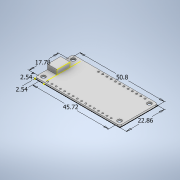
# Autodesk Inventor part: Adafruit Feather 32u4
Saved by Autodesk Inventor 2020.2 (Build 242310000, 310)
## iProperties
Created: 2019-11-22
Part Number: Adafruit Feather 32u4
Material: Generic
Document SubType Name: Sheet Metal
Designer: athiy
Density: 1 g/cm^3
Sheet Metal Rule: Default
Appearance: Default
Author: athiy
Autodesk Inventor part; units mm, degrees
ref_plane "YZ Plane" through (0, 0, 0) normal (1, 0, 0) x (0, 1, 0)
ref_plane "XZ Plane" through (0, 0, 0) normal (0, 1, 0) x (-1, 0, 0)
ref_plane "XY Plane" through (0, 0, 0) normal (0, 0, 1) x (1, 0, 0)
sketch "Sketch1" plane through (0, 0, 0) normal (0, 1, 0) x (-1, 0, 0)
  line L0 (0, 0) -> (-50.8, 0)
  line L1 (-50.8, 0) -> (-50.8, -22.86)
  line L2 (-50.8, -22.86) -> (0, -22.86)
  line L3 (0, -22.86) -> (0, 0)
  line L4 (0, 0) -> (-2.54, 0)
  line L5 (-2.54, 0) -> (-48.26, 0)
  line L6 (0, 0) -> (0, -2.54)
  line L7 (0, -2.54) -> (0, -20.32)
  dimension "d0" = 50.8
  dimension "d1" = 22.86
  dimension "d2" = 2.54
  dimension "d3" = 45.72
  dimension "d4" = 2.54
  dimension "d5" = 17.78
  constraints: 16 end point, 4 point on line, 2 parallel, 1 horizontal, 1 perpendicular
  measures "d0" distance of L2.end L1.end
  measures "d1" distance of L1.end L0.end
  measures "d2" distance of L0.start L4.end
  measures "d3" distance of L4.end L5.end
  measures "d4" distance of L0.start L6.end
  measures "d5" distance of L6.end L7.end
sketch "Sketch2" plane through (0, 0, 0) normal (0, 1, 0) x (-1, 0, 0)
  point P0 (0, 0)
sketch "Sketch3" plane through (0, 0, 0) normal (0, 1, 0) x (-1, 0, 0)
  line L0 (0, -1.27) -> (0, -1.27)
  line L1 (0, -2.504) -> (-2.54, -2.504)
  line L2 (-2.54, -2.504) -> (-2.54, 0)
  line L3 (0, -11.43) -> (-50.8, -11.43)
  circle A0 centre (-2.54, -2.504) radius 1.27
  circle A1 centre (-2.54, -20.356) radius 1.27
  line L4 (-25.4, 0) -> (-25.4, -22.86)
  circle A2 centre (-48.26, -2.504) radius 1.27
  circle A3 centre (-48.26, -20.356) radius 1.27
  line L5 (-1.27, 0) -> (-1.27, 0)
  arc A4 (0, -1.27) -> (-1.27, 0) centre (-1.27, -1.27) ccw
  arc A5 (-1.27, -22.86) -> (0, -21.59) centre (-1.27, -21.59) ccw
  arc A6 (-49.53, 0) -> (-50.8, -1.27) centre (-49.53, -1.27) ccw
  arc A7 (-50.8, -21.59) -> (-49.53, -22.86) centre (-49.53, -21.59) ccw
  line L6 (-25.4, -1.27) -> (-6.35, -1.27)
  line L7 (-25.4, -1.27) -> (-44.45, -1.27)
  circle A8 centre (-6.35, -1.27) radius 0.51
  line L8 (-6.35, -1.27) -> (-8.89, -1.27)
  line L9 (-6.35, -1.27) -> (-3.81, -1.27) construction
  circle A9 centre (-8.89, -1.27) radius 0.51
  circle A10 centre (-8.89, -1.27) radius 0.51
  circle A11 centre (-11.43, -1.27) radius 0.51
  circle A12 centre (-13.97, -1.27) radius 0.51
  circle A13 centre (-16.51, -1.27) radius 0.51
  circle A14 centre (-19.05, -1.27) radius 0.51
  circle A15 centre (-21.59, -1.27) radius 0.51
  circle A16 centre (-24.13, -1.27) radius 0.51
  circle A17 centre (-44.45, -1.27) radius 0.51
  circle A18 centre (-41.91, -1.27) radius 0.51
  circle A19 centre (-39.37, -1.27) radius 0.51
  circle A20 centre (-36.83, -1.27) radius 0.51
  circle A21 centre (-34.29, -1.27) radius 0.51
  circle A22 centre (-31.75, -1.27) radius 0.51
  circle A23 centre (-29.21, -1.27) radius 0.51
  circle A24 centre (-26.67, -1.27) radius 0.51
  circle A25 centre (-16.51, -21.59) radius 0.51
  circle A26 centre (-19.05, -21.59) radius 0.51
  circle A27 centre (-21.59, -21.59) radius 0.51
  circle A28 centre (-24.13, -21.59) radius 0.51
  circle A29 centre (-29.21, -21.59) radius 0.51
  circle A30 centre (-26.67, -21.59) radius 0.51
  circle A31 centre (-31.75, -21.59) radius 0.51
  circle A32 centre (-34.29, -21.59) radius 0.51
  circle A33 centre (-36.83, -21.59) radius 0.51
  circle A34 centre (-39.37, -21.59) radius 0.51
  circle A35 centre (-41.91, -21.59) radius 0.51
  circle A36 centre (-44.45, -21.59) radius 0.51
  line L10 (-1.27, -22.86) -> (-49.53, -22.86)
  line L11 (-50.8, -21.59) -> (-50.8, -1.27)
  line L12 (-49.53, 0) -> (-1.27, 0)
  line L13 (0, -1.27) -> (0, -21.59)
  point P0 (0, 0)
  dimension "d11" = 22.86
  dimension "d12" = 1.27
  dimension "d13" = 19.05
  dimension "d18" = 1.02
  dimension "d19" = 2.54
  dimension "d20" = 180
  dimension "d21" = 1.02
  dimension "d24" = 2.54
  dimension "d31" = 2.54
  dimension "d38" = 2.54
  constraints: 37 centre point, 33 symmetric about line, 28 end point, 8 horizontal, 8 point on circle, 4 perpendicular, 3 point on line, 3 tangent, 2 coincident, 2 collinear, 2 vertical, 40 other
  measures "d11" distance of L4.start L4.end
  measures "d12" radius of A4
  measures "d13" distance of L6.start L6.end
  measures "d18" diameter of A8
  measures "d19" distance of L8.start L8.end
  measures "d20" angle of L8 L9
  measures "d21" diameter of A9
  measures "d24" distance of L8.start A10.centre
  measures "d31" distance of A11.centre A12.centre
  measures "d38" distance of A15.centre A16.centre
sketch "Sketch4" plane through (0, 0, 0) normal (0, 1, 0) x (-1, 0, 0)
  point P0 (0, 0)
extrude "Extrusion1" add sketch "Sketch3" along normal blind 1.016 contours L13 L3 L4 L12 L2 A0 L1 | L1 A0 L2 L12 A4 L13 | L13 A5 L10 L4 L3 | L4 L10 A7 L11 L3 | L3 L11 A6 L12 L4
sketch "Sketch5" plane through (0, 1.016, 0) normal (0, 1, 0) x (1, 0, 0)
  line L0 (0, 21.59) -> (0, 1.27) projected
  line L1 (0, 11.43) -> (0, 15.38)
  line L2 (0, 15.38) -> (5.6, 15.38)
  line L3 (5.6, 15.38) -> (5.6, 7.48)
  line L4 (5.6, 7.48) -> (0, 7.48)
  point P0 (0, 0)
  dimension "d46" = 3.95
  dimension "d49" = 5.6
  dimension "d50" = 7.9
  constraints: 8 end point, 2 perpendicular, 2 point on line, 1 horizontal, 1 midpoint
  measures "d46" distance of L1.start L1.end
  measures "d49" distance of L1.end L2.end
  measures "d50" distance of L2.end L3.end
extrude "Extrusion2" add sketch "Sketch5" along normal blind 2.8
sketch "Sketch6" plane through (5.6, 1.016, -7.48) normal (1, 0, 0) x (0, 0, -1)
  line L0 (0, 0) -> (0, 2.8) projected
  line L1 (7.9, 2.8) -> (0, 2.8) projected
  line L2 (7.9, 0) -> (7.9, 2.8) projected
  line L3 (-6.21, 0) -> (14.11, 0) projected
  point P0 (-7.48, -1.016)
sketch "Sketch7" plane through (0, 0, -21.59) normal (-1, 0, 0) x (0, 0, 1)
  line L0 (6.21, 3.816) -> (6.51, 3.816)
  line L1 (6.51, 3.216) -> (13.81, 3.216)
  line L2 (13.81, 3.216) -> (13.81, 1.316)
  line L3 (13.81, 1.316) -> (6.51, 1.316)
  line L4 (6.51, 1.316) -> (6.51, 3.216)
  point P0 (21.59, 0)
  dimension "d61" = 0.3
  dimension "d62" = 0.6
  dimension "d63" = 7.3
  dimension "d64" = 1.9
  constraints: 10 end point, 3 perpendicular
  measures "d61" distance of L0.start L0.end
  measures "d62" distance of L0.end L1.start
  measures "d63" distance of L1.start L1.end
  measures "d64" distance of L1.end L2.end
sketch "Sketch8" plane through (5.6, 1.016, -7.48) normal (1, 0, 0) x (0, 0, -1)
  point P0 (-7.48, -1.016)
extrude "Extrusion3" cut sketch "Sketch7" against normal blind 2.15
equation "\"BendRadius\" = Thickness"
equation "\"BendReliefWidth\" = Thickness"
equation "\"BendReliefDepth\" = 0.5 * Thickness"
equation "\"CornerReliefSize\" = 4 * Thickness"
equation "\"MinimumRemnant\" = 2 * Thickness"
equation "\"TransitionRadius\" = BendRadius"
equation "\"JacobiRadiusSize\" = Thickness"
equation "\"GapSize\" = Thickness"
equation "\"Thickness\" = 0.5"
body "Solid1"
